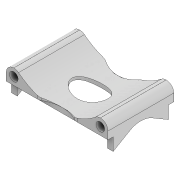
# Autodesk Inventor part: oxybeamTop
Saved by Autodesk Inventor 2020 (Build 240168000, 168)
## iProperties
Created: 2020-05-15
Part Number: oxybeamTop
Material: Generic
Document SubType Name: Modeling
Designer: rayan
Density: 1 g/cm^3
Appearance: Default
Author: rayan
Autodesk Inventor part; units mm, degrees
ref_plane "XZ Plane" through (0, 0, 0) normal (0, 1, 0) x (-1, 0, 0)
ref_plane "XY Plane" through (0, 0, 0) normal (0, 0, 1) x (1, 0, 0)
sketch "Sketch1" plane through (0, 0, 0) normal (0, 0, 1) x (1, 0, 0)
  circle A0 centre (0, 0) radius 1.7
  circle A1 centre (0, 0) radius 3
  dimension "d0" = 3.4
  dimension "d1" = 6
  constraints: 2 centre point, 2 coincident
  measures "d0" diameter of A0
  measures "d1" diameter of A1
extrude "Extrusion1" add sketch "Sketch1" along normal mid plane 26
sketch "Sketch2" plane through (0, 0, 13) normal (0, 0, 1) x (1, 0, 0)
  circle A0 centre (0, 0) radius 1.7 projected
  circle A1 centre (0, 0) radius 3 construction
  line L0 (-3, 0) -> (-0.7, 0)
  line L1 (-0.7, 0) -> (-0.7, -8)
  line L2 (-0.7, -8) -> (-3, -8)
  line L3 (-3, -8) -> (-3, 0)
  line L4 (3, 0) -> (-0.7, 0)
  line L5 (-0.7, 0) -> (-0.7, -5)
  line L6 (-0.7, -5) -> (3, -5)
  line L7 (3, -5) -> (3, 0)
  line L8 (-0.7, -5) -> (-0.7, -8)
  line L9 (-3, 0) -> (-1.85, 0)
  line L10 (1.7, 0) -> (3, 0)
  point P0 (-1.7, 0)
  dimension "d19" = 2.3
  dimension "d20" = 8
  dimension "d21" = 5
  constraints: 22 end point, 4 parallel, 3 perpendicular, 2 horizontal, 2 point on circle, 1 collinear, 1 midpoint, 1 point on line, 2 other
  measures "d19" distance of L1.end L2.end
  measures "d20" distance of L0.end L1.end
  measures "d21" distance of L5.end L0.end
extrude "Extrusion2" add sketch "Sketch2" against normal up to surface (26 mm away) contours L4 L7 L6 L1 A0 | A0 L1 L2 L3 L0
sketch "Sketch3" plane through (0, 0, 13) normal (0, 0, 1) x (1, 0, 0)
  line L0 (3, -5) -> (3, 0) projected
  line L1 (-3, -8) -> (3, -8)
  line L2 (3, -8) -> (3, -3)
  line L3 (3, -3) -> (-3, -3)
  line L4 (-3, -3) -> (-3, -8)
  point P0 (0, 0)
  dimension "d10" = 5
  constraints: 8 end point, 2 parallel, 1 horizontal, 1 perpendicular, 1 point on line
  measures "d10" distance of L2.end L1.end
extrude "Extrusion3" cut sketch "Sketch3" against normal blind 2.05
mirror "Mirror1" about plane through (0, 0, 0) normal (0, 0, 1) of "Extrusion3"
sketch "Sketch5" plane through (-3, 0, -13) normal (-1, 0, 0) x (0, 0, 1)
  line L0 (2.05, -8) -> (2.05, -5) projected
  line L1 (2.05, -8) -> (5.05, -8)
  line L2 (23.95, -8) -> (2.05, -8) projected
  line L3 (2.05, -8) -> (5.05, -8) construction
  line L4 (23.95, -8) -> (20.95, -8)
  line L5 (23.95, -8) -> (26.95, -8) construction
  line L6 (2.05, -3) -> (23.95, -3)
  arc A0 (20.95, -8) -> (5.05, -8) centre (13, -11.8202) ccw
  point P0 (13, 0)
  dimension "d22" = 3
  dimension "d23" = 0
  dimension "d24" = 3
  dimension "d25" = 180
  constraints: 10 end point, 4 collinear, 3 horizontal, 2 point on circle, 1 centre point, 1 tangent
  measures "d22" distance of L0.start L1.end
  measures "d23" distance between parallel lines of L1 L3
  measures "d24" distance of L2.start L4.end
  measures "d25" angle of L4 L5
extrude "Extrusion5" cut sketch "Sketch5" against normal through all
fillet "Fillet3" radius 200 2 edges at (-1.85, -8, -7.95) (-1.85, -8, 7.95)
ref_plane "Work Plane1" through (17.1, 0, 0) normal (1, 0, 0) x (0, 1, 0)
mirror "Mirror2" about plane through (17.1, 0, 0) normal (1, 0, 0) of "Extrusion1", "Extrusion2", "Extrusion3", "Mirror1", "Extrusion5", "Fillet3"
sketch "Sketch7" plane through (3, 0, 13) normal (1, 0, 0) x (0, 0, -1)
  arc A0 (7.2315, -5) -> (8.4146, -4.2856) centre (-95.5595, 166.5634) ccw projected
  arc A1 (17.5854, -4.2856) -> (8.4146, -4.2856) centre (13, -11.8202) ccw projected
  arc A2 (17.5854, -4.2856) -> (18.7685, -5) centre (121.5595, 166.5634) ccw projected
  line L0 (18.7685, -5) -> (23.95, -5) projected
  line L1 (23.95, -5) -> (23.95, -3) projected
  line L2 (23.95, -3) -> (26, -3) projected
  line L3 (26, 0) -> (26, -3) projected
  line L4 (26, 0) -> (0, 0) projected
  line L5 (0, -3) -> (0, 0) projected
  line L6 (0, -3) -> (2.05, -3) projected
  line L7 (2.05, -3) -> (2.05, -5) projected
  line L8 (2.05, -5) -> (7.2315, -5) projected
  line L9 (26, -3) -> (26, 0) projected
  line L10 (26, 0) -> (0, 0)
  line L11 (0, 0) -> (0, -1.5)
  line L12 (0, -1.5) -> (26, -1.5)
  line L13 (26, -1.5) -> (26, 0)
  point P0 (13, 0)
  point P1 (0, -1.5)
  dimension "d32" = 1.5
  constraints: 8 end point, 3 equal length, 1 perpendicular
  measures "d32" distance between parallel lines of L6 L12
extrude "Extrusion7" add sketch "Sketch7" along normal up to surface (28.2 mm away) contours L8 L7 L6 L5 L12 L3 L2 L1 L0 A2 A1 A0
sketch "Sketch8" plane through (3, -1.5, 13) normal (0, 1, 0) x (1, 0, 0)
  line L0 (28.2, 26) -> (28.2, 0) construction
  line L1 (0, 26) -> (28.2, 26) construction
  line L2 (0, 0) -> (0, 26) construction
  line L3 (0, 0) -> (28.2, 0) construction
  line L4 (0, 26) -> (28.2, 26) construction
  line L5 (0, 0) -> (28.2, 26) construction
  line L6 (-3.7, 18.7685) -> (31.9, 18.7685) projected
  line L7 (0, 0) -> (0, 26) projected
  line L8 (28.2, 7.2315) -> (0, 7.2315)
  line L9 (0, 7.2315) -> (0, 18.7685)
  line L10 (0, 18.7685) -> (28.2, 18.7685)
  line L11 (28.2, 18.7685) -> (28.2, 7.2315)
  line L12 (28.2, 7.2315) -> (0, 18.7685) construction
  line L13 (0, 7.2315) -> (28.2, 18.7685) construction
  point P0 (-3, 13)
  point P1 (14.1, 13)
  point P2 (0, 7.2315)
  constraints: 14 end point, 3 midpoint, 2 parallel, 2 point on line, 1 horizontal, 1 perpendicular
extrude "Extrusion8" [suppressed]
fillet "Fillet4" radius 1.5 2 edges at (31.2, -1.5, 0) (3, -1.5, 0)
fillet "Fillet5" [suppressed]
sketch "Sketch9" plane through (0, 0, 13) normal (0, 0, 1) x (1, 0, 0)
  arc A0 (3, 0) -> (-3, 0) centre (0, 0) ccw construction
  line L0 (0, 0) -> (0, 3)
  line L1 (0, 3) -> (1.1, 3)
  line L2 (1.1, 3) -> (1.1, 0) construction
  line L3 (1.1, 0) -> (0, 0) construction
  circle A1 centre (34.2, 0) radius 1.7 construction
  arc A2 (37.2, 0) -> (31.2, 0) centre (34.2, 0) ccw construction
  line L4 (34.2, 0) -> (34.2, 3)
  line L5 (34.2, 3) -> (33.1, 3)
  line L6 (33.1, 3) -> (33.1, 0) construction
  line L7 (33.1, 0) -> (34.2, 0) construction
  line L8 (0, 0) -> (34.2, 0) construction
  line L9 (34.2, 0) -> (34.2, -3)
  line L10 (34.2, -3) -> (0, -3)
  line L11 (0, -3) -> (0, 0)
  arc A3 (1.1, 3) -> (33.1, 3) centre (17.1, 21.3333) ccw
  circle A4 centre (34.2, 0) radius 1.7 projected
  line L12 (-3, -3) -> (37.2, -3) projected
  line L13 (37.2, 0) -> (37.2, -3) projected
  arc A5 (37.2, 0) -> (31.2, 0) centre (34.2, 0) ccw construction
  arc A6 (29.7, -1.5) -> (31.2, 0) centre (29.7, 0) ccw construction
  line L14 (4.5, -1.5) -> (29.7, -1.5) construction
  arc A7 (3, 0) -> (4.5, -1.5) centre (4.5, 0) ccw construction
  arc A8 (3, 0) -> (-3, 0) centre (0, 0) ccw construction
  line L15 (-3, 0) -> (-3, -3) projected
  circle A9 centre (0, 0) radius 1.7 projected
  line L16 (5.3953, 0) -> (28.8047, 0)
  point P0 (17.1, -3)
  point P1 (0, 1.7)
  point P2 (0, -1.7)
  point P3 (34.2, -1.7)
  point P4 (34.2, 1.7)
  dimension "d39" = 1.1
  dimension "d40" = 1.1
  dimension "d41" = 3
  constraints: 26 end point, 7 point on circle, 6 parallel, 4 perpendicular, 3 point on line, 1 centre point, 1 midpoint, 1 vertical
  measures "d39" distance of L0.end L1.end
  measures "d40" distance of L5.end L4.end
  measures "d41" distance of L8.end L9.end
extrude "Extrusion9" add sketch "Sketch9" against normal up to surface (26 mm away) contours L0 L1 A3 L10 L11 A9 | A3 L5 L4 A4 L9 L10
extrude "Extrusion10" cut sketch "Sketch9" against normal through all contours A3 L16
fillet "Fillet6" radius 3 2 edges at (33.1, 3, 0) (1.1, 3, 0)
sketch "Sketch10" plane through (37.2, -3, 10.95) normal (0, -1, 0) x (1, 0, 0)
  line L0 (-38.9, 2.05) -> (-35.5, 2.05) construction
  line L1 (-1.3, 2.05) -> (-4.7, 2.05) construction
  line L2 (-37.2, 2.05) -> (-27.2, 2.05) construction
  line L3 (-40.2, 2.05) -> (-20.1, 2.05) construction
  line L4 (-3, 2.05) -> (-3.012, 2.05) construction
  line L5 (-3.012, 2.05) -> (-13.012, 2.05) construction
  line L6 (-20.1, 2.05) -> (-20.1, 0) construction
  arc A0 (-27.2, 2.05) -> (-13.012, 2.05) centre (-20.106, 13.2994) ccw
  line L7 (-27.2, 2.05) -> (-13.012, 2.05) construction
  line L8 (-20.1, 2.05) -> (0, 2.05) construction
  line L9 (-20.1, -21.9) -> (-20.1, -23.95) construction
  line L10 (-40.2, -21.9) -> (-20.1, -21.9) construction
  line L11 (-40.2, -23.95) -> (-40.2, -21.9) projected
  line L12 (-20.1, -23.95) -> (-40.2, -23.95) construction
  line L13 (0, -23.95) -> (-20.1, -23.95) construction
  line L14 (0, -21.9) -> (0, -23.95) projected
  line L15 (-20.1, -21.9) -> (0, -21.9) construction
  line L16 (-27.2, 2.05) -> (-13.012, 2.05) construction
  line L17 (-13.012, 2.05) -> (-13.012, -23.95) construction
  line L18 (-13.012, -23.95) -> (-27.2, -23.95) construction
  line L19 (-27.2, -23.95) -> (-27.2, 2.05) construction
  arc A1 (-13.012, -23.95) -> (-27.2, -23.95) centre (-20.106, -35.1994) ccw
  line L20 (-27.2, 2.05) -> (-13.012, -23.95) construction
  line L21 (-20.106, -10.95) -> (-27.2, -10.95) construction
  ellipse E0 centre (-20.106, -10.95) end of major axis (-27.2, -10.95) minor radius 5
  line L22 (-27.2, 2.05) -> (-13.012, 2.05)
  line L23 (-20.1, 2.05) -> (-4.8875, 2.05) projected
  line L24 (-27.2, -23.95) -> (-13.012, -23.95)
  line L25 (-4.8875, -23.95) -> (-20.1, -23.95) projected
  point P0 (-37.2, -10.95)
  dimension "d50" = 5
  dimension "d47" = 10
  dimension "d48" = 10
  dimension "d49" = 26
  constraints: 22 end point, 6 point on circle, 4 collinear, 3 midpoint, 2 centre point, 2 horizontal, 2 parallel, 1 coincident, 1 horizontal alignment, 1 perpendicular, 1 point on line, 2 other
  measures "d47" distance of L2.start L2.end
  measures "d48" distance of L4.end L5.end
  measures "d49" distance of L5.end L17.end
extrude "Extrusion11" cut sketch "Sketch10" against normal through all both and the other way through all
fillet "Fillet7" radius 3 4 edges at (24.188, -2.4724, 13) (10, -2.4706, 13) (10, -2.4706, -13) (24.188, -2.4724, -13)
equation "\"d48\" = d47"
body "Solid1"
